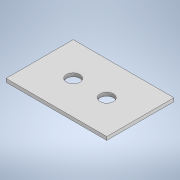
# Autodesk Inventor part: trail 10
Saved by Autodesk Inventor 2020.2 (Build 242310000, 310)
## iProperties
Created: 2020-02-17
Part Number: trail 10
Material: Generic
Document SubType Name: Modeling
Designer: lenovo
Density: 1 g/cm^3
Appearance: Default
Author: lenovo
Autodesk Inventor part; units mm, degrees
ref_plane "YZ Plane" through (0, 0, 0) normal (1, 0, 0) x (0, 1, 0)
ref_plane "XZ Plane" through (0, 0, 0) normal (0, 1, 0) x (-1, 0, 0)
ref_plane "XY Plane" through (0, 0, 0) normal (0, 0, 1) x (1, 0, 0)
sketch "Sketch1" plane through (0, 0, 0) normal (0, 1, 0) x (-1, 0, 0)
  line L0 (-15, -10) -> (15, -10)
  line L1 (15, -10) -> (15, 10)
  line L2 (15, 10) -> (-15, 10)
  line L3 (-15, 10) -> (-15, -10)
  line L4 (-15, -10) -> (15, 10) construction
  line L5 (15, -10) -> (-15, 10) construction
  circle A0 centre (5, 0) radius 2
  circle A1 centre (-5, 0) radius 2
  point P0 (0, 0)
  dimension "d0" = 30
  dimension "d1" = 20
  dimension "d2" = 4
  dimension "d3" = 4
  constraints: 12 end point, 2 centre point, 2 midpoint, 2 parallel, 1 horizontal, 1 perpendicular
  measures "d0" distance of L2.end L1.end
  measures "d1" distance of L1.end L0.end
  measures "d2" diameter of A0
  measures "d3" diameter of A1
extrude "Extrusion1" add sketch "Sketch1" along normal blind 1
body "Solid1"
